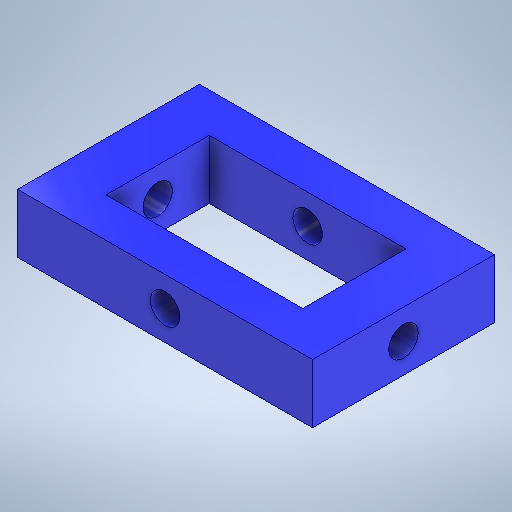
# Autodesk Inventor part: Shifter Joint 2
Saved by Autodesk Inventor 2025.2 (Build 292293000, 293)
## iProperties
Created: 2025-02-09
Part Number: Shifter Joint 2
Material: Generic
Document SubType Name: Modeling
Designer: eason
Density: 1 g/cm^3
Appearance: Blue - Wall Paint - Glossy
Author: eason
Autodesk Inventor part; units mm, degrees
ref_plane "YZ Plane" through (0, 0, 0) normal (1, 0, 0) x (0, 1, 0)
ref_plane "XZ Plane" through (0, 0, 0) normal (0, 1, 0) x (-1, 0, 0)
ref_plane "XY Plane" through (0, 0, 0) normal (0, 0, 1) x (1, 0, 0)
sketch "Sketch1" plane through (0, 0, 0) normal (0, 0, 1) x (1, 0, 0)
  circle A0 centre (0, 0) radius 3
  circle A1 centre (0, 0) radius 6
  line L0 (-30, 6) -> (0, 6)
  line L1 (-30, -6) -> (0, -6)
  line L2 (-30, 6) -> (-30, -6)
  line L3 (0, -8.4) -> (0, 8.4) projected
  line L4 (30, 6) -> (0, 6)
  line L5 (30, -6) -> (0, -6)
  line L6 (30, 6) -> (30, -6)
  dimension "d0" = 6
  dimension "d1" = 3
  dimension "d2" = 30
  constraints: 12 end point, 2 centre point, 2 coincident, 2 horizontal, 2 point on circle, 2 symmetric about line, 2 tangent, 1 parallel, 1 vertical
  measures "d0" diameter of A0
  measures "d1" radial gap between concentric circles of A0 A1
  measures "d2" distance between parallel lines of L3 L2
extrude "Extrusion1" add sketch "Sketch1" along normal blind 8 contours A0 L3 A1 | A0 L3 A1 | L4 L6 L5 A1 | A1 L1 L2 L0
sketch "Sketch2" plane through (0, 0, 0) normal (0, 0, 1) x (1, 0, 0)
  line L0 (30, 6) -> (-30, 6) projected
  line L1 (-30, 6) -> (-20, 6)
  line L2 (-20, 6) -> (-20, -6)
  line L3 (-20, -6) -> (-30, -6)
  line L4 (-30, -6) -> (-30, 6)
  line L5 (-30, -6) -> (30, -6) projected
  line L6 (30, -6) -> (30, 6) projected
  line L7 (30, 6) -> (20, 6)
  line L8 (20, 6) -> (20, -6)
  line L9 (20, -6) -> (30, -6)
  line L10 (30, -6) -> (30, 6)
  point P0 (0, 0)
  point P1 (20, 6)
  dimension "d5" = 10
  dimension "d6" = 10
  constraints: 16 end point, 4 parallel, 2 horizontal, 2 perpendicular, 1 collinear, 1 point on line
  measures "d5" distance between parallel lines of L4 L2
  measures "d6" distance between parallel lines of L6 L8
extrude "Extrusion2" add sketch "Sketch2" against normal blind 21 contours L6 L5 L8 L0 | L2 L3 L4 L0
sketch "Sketch3" plane through (0, 0, -21) normal (0, 0, -1) x (-1, 0, 0)
  line L0 (-30, -6) -> (-30, 6) projected
  line L1 (30, -6) -> (-30, -6) projected
  line L2 (-30, 6) -> (30, 6)
  line L3 (30, 6) -> (30, -6)
  line L4 (30, -6) -> (-30, -6)
  line L5 (-30, -6) -> (-30, 6)
  point P0 (0, 0)
  constraints: 8 end point, 2 parallel, 1 horizontal, 1 perpendicular
extrude "Extrusion3" add sketch "Sketch3" along normal blind 8
extrude "Extrusion4" cut sketch "Sketch1" against normal through all contours A0 L3 | L3 A0
sketch "Sketch4" plane through (-30, -6, 8) normal (-1, 0, 0) x (0, 0, 1)
  circle A0 centre (-18.5, 6) radius 3
  line L0 (-37, 0) -> (-37, 12) projected
  line L1 (-37, 12) -> (0, 0) construction
  line L2 (-37, 12) -> (0, 12) projected
  line L3 (0, 12) -> (-37, 0) construction
  point P0 (-8, 6)
  dimension "d13" = 6
  constraints: 4 end point, 2 coincident, 1 centre point, 1 midpoint
  measures "d13" diameter of A0
extrude "Extrusion5" cut sketch "Sketch4" against normal through all
body "Solid1"
